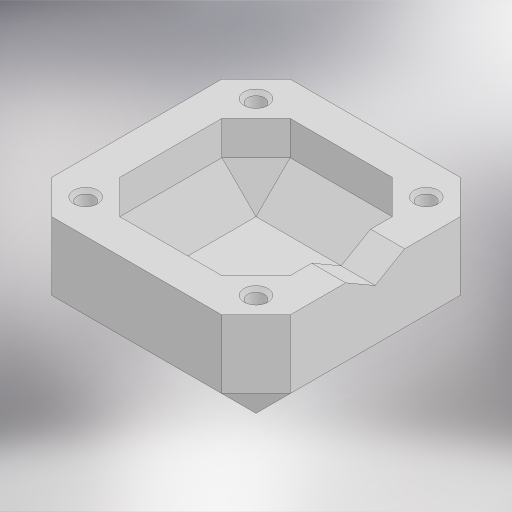
# Autodesk Inventor part: pokemon_ball_white
Saved by Autodesk Inventor 2024 (Build 280153000, 153)
## iProperties
Created: 2023-10-25
Part Number: pokemon_ball_white
Material: Generic
Document SubType Name: Modeling
Designer: SSAFY
Density: 1 g/cm^3
Appearance: Default
Author: SSAFY
Autodesk Inventor part; units mm, degrees
ref_plane "YZ Plane" through (0, 0, 0) normal (1, 0, 0) x (0, 1, 0)
ref_plane "XZ Plane" through (0, 0, 0) normal (0, 1, 0) x (-1, 0, 0)
ref_plane "XY Plane" through (0, 0, 0) normal (0, 0, 1) x (1, 0, 0)
sketch "Sketch2" plane through (0, 0, 0) normal (0, 1, 0) x (-1, 0, 0)
  line L0 (25, -25) -> (-25, -25)
  line L1 (-25, -25) -> (-25, 25)
  line L2 (-25, 25) -> (25, 25)
  line L3 (25, 25) -> (25, -25)
  line L4 (25, -25) -> (-25, 25) construction
  line L5 (-25, -25) -> (25, 25) construction
  line L6 (35, 35) -> (-35, 35)
  line L7 (-35, 35) -> (-35, -35)
  line L8 (-35, -35) -> (35, -35)
  line L9 (35, -35) -> (35, 35)
  point P0 (0, 0)
  dimension "d0" = 50
  dimension "d1" = 10
  dimension "d19" = 50
  constraints: 20 end point, 4 parallel, 2 midpoint, 2 perpendicular, 1 horizontal, 3 other
  measures "d0" distance of L1.end L2.end
  measures "d1" distance between parallel lines of L2 L6
  measures "d19" distance of L2.end L0.start
extrude "Extrusion1" add sketch "Sketch2" along normal mid plane 30
sketch "Sketch3" plane through (0, -15, 0) normal (0, -1, 0) x (1, 0, 0)
  line L0 (35, -35) -> (35, 35) projected
  line L1 (35, 35) -> (-35, 35) projected
  line L2 (-35, 35) -> (-35, -35) projected
  line L3 (-35, -35) -> (35, -35) projected
  point P0 (0, 0)
extrude "Extrusion2" add sketch "Sketch3" against normal blind 10
chamfer "Chamfer1" distance 10 angle 45 16 edges at (35, 0, 35) (25, 5, 25) (-25, 5, 25) (-35, 0, 35) (-25, 5, -25) (25, 5, -25) (-35, 0, -35) (35, 0, -35) (0, -5, -25) (25, -5, 0) (0, -5, 25) (-25, -5, 0) (0, -15, -35) (35, -15, 0) (0, -15, 35) (-35, -15, 0)
sketch "Sketch4" plane through (35, -5, -25) normal (1, 0, 0) x (0, 0, -1)
  line L0 (0, 20) -> (0, 0) construction
  line L1 (-50, 20) -> (0, 20) construction
  line L2 (-16.3397, 30) -> (-16.3397, 20)
  line L3 (-16.3397, 20) -> (-25, 15)
  line L4 (-25, 15) -> (-33.6603, 20)
  line L5 (-33.6603, 20) -> (-33.6603, 30)
  line L6 (-33.6603, 30) -> (-25, 35)
  line L7 (-25, 35) -> (-16.3397, 30)
  point P0 (-25, 5)
  point P1 (-25, 25)
  dimension "d9" = 10
  dimension "d10" = 5
  dimension "d20" = 0
  constraints: 12 end point, 1 parallel, 13 other
  measures "d9" distance of L4.end L5.end
  measures "d10" distance from line of point (-25, 25) L1
  measures "d20" horizontal distance of point (-25, 5) point (-25, 25)
extrude "Extrusion3" cut sketch "Sketch4" against normal blind 10
sketch "Sketch5" plane through (0, 15, 0) normal (0, 1, 0) x (1, 0, 0)
  line L0 (-25, 25) -> (-25, 35) construction
  circle A0 centre (-25, 25) radius 2.5
  line L1 (25, 25) -> (35, 25) construction
  circle A1 centre (25, 25) radius 2.5
  line L2 (-25, -25) -> (-35, -25) construction
  circle A2 centre (-25, -25) radius 2.5
  line L3 (-25, -25) -> (25, -25) construction
  circle A3 centre (25, -25) radius 2.5
  point P0 (0, 0)
  dimension "d13" = 5
  dimension "d14" = 5
  dimension "d15" = 5
  dimension "d16" = 5
  constraints: 4 centre point, 1 end point
  measures "d13" diameter of A0
  measures "d14" diameter of A2
  measures "d15" diameter of A1
  measures "d16" diameter of A3
extrude "Extrusion4" cut sketch "Sketch5" against normal blind 10
chamfer "Chamfer2" distance 1 angle 45 4 edges at (-27.5, 15, 25) (-27.5, 15, -25) (22.5, 15, 25) (22.5, 15, -25)
body "Solid1"
